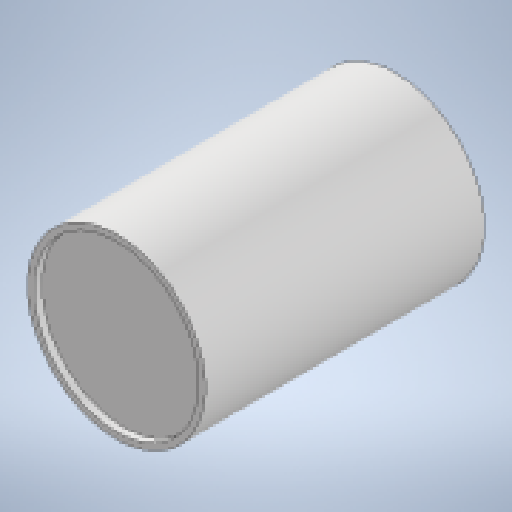
# Autodesk Inventor part: GrundkörperOben
Saved by Autodesk Inventor 2024 (Build 280153000, 153)
## iProperties
Created: 2024-02-13
Part Number: GrundkörperOben
Material: Generic
Document SubType Name: Modeling
Designer: Daniel Nussbaum
Density: 1 g/cm^3
Appearance: Default
Author: Daniel Nussbaum
Autodesk Inventor part; units mm, degrees
ref_plane "YZ Plane" through (0, 0, 0) normal (1, 0, 0) x (0, 1, 0)
ref_plane "XZ Plane" through (0, 0, 0) normal (0, 1, 0) x (-1, 0, 0)
ref_plane "XY Plane" through (0, 0, 0) normal (0, 0, 1) x (1, 0, 0)
sketch "Sketch1" plane through (0, 0, 0) normal (0, 1, 0) x (-1, 0, 0)
  line L0 (-67.5, -60) -> (-67.5, 0)
  line L1 (2.5, -60) -> (2.5, 0)
  line L2 (-67.5, 0) -> (2.5, 0)
  line L3 (-32.5, 0) -> (-32.5, 110)
  line L4 (2.5, -60) -> (-67.5, -60) projected
  line L5 (-67.5, 0) -> (-67.5, 110)
  line L6 (-65, 0) -> (-65, -30)
  line L7 (0, 0) -> (0, -30)
  line L8 (-65, 0) -> (-65, 110)
  line L9 (-65, 110) -> (-67.5, 110)
  line L10 (-65, 0) -> (-67.5, 0)
  line L11 (-65, 107) -> (-32.5, 107)
  line L12 (-32.5, 107) -> (-32.5, 102)
  line L13 (-32.5, 102) -> (-65, 102)
  line L14 (-65, 102) -> (-65, 107)
  dimension "d1" = 170
  dimension "d2" = 5
  dimension "d3" = 3
  constraints: 28 end point, 7 vertical, 3 parallel, 2 horizontal, 2 perpendicular, 2 point on line, 1 midpoint, 7 other
  measures "d1" distance from line of L3.end L4
  measures "d2" distance between parallel lines of L11 L13
  measures "d3" distance between parallel lines of L9 L11
revolve "Revolution1" add sketch "Sketch1" angle 360 about axis through (32.5, 0, 0) along (0, 0, 1) contours L5 L9 L8 L2 | L8 L11 L3 L13
sketch "Sketch2" plane through (0, 0, 0) normal (0, 1, 0) x (-1, 0, 0)
  line L0 (2.5, 0) -> (-67.5, 0) projected
  line L1 (2.5, 110) -> (-67.5, 110) projected
  line L2 (-32.5, 0) -> (-32.5, 5)
  circle A0 centre (-32.5, 5) radius 1.5
  point P0 (0, 0)
  dimension "d5" = 5
  dimension "d6" = 3
  constraints: 2 end point, 1 centre point, 1 coincident, 1 midpoint, 1 vertical
  measures "d5" distance of L2.start L2.end
  measures "d6" diameter of A0
extrude "Extrusion1" cut sketch "Sketch2" along normal through all both and the other way through all
sketch "Sketch3" plane through (0, 0, 0) normal (1, 0, 0) x (0, 1, 0)
  line L0 (35, 0) -> (-35, 0) projected
  line L1 (35, 110) -> (-35, 110) projected
  line L2 (0, 0) -> (0, 5)
  circle A0 centre (0, 5) radius 1.5
  point P0 (34.9678, 5)
  point P1 (-34.9678, 5)
  dimension "d9" = 5
  dimension "d10" = 3
  constraints: 2 end point, 1 centre point, 1 coincident, 1 vertical
  measures "d9" distance of L2.start L2.end
  measures "d10" diameter of A0
extrude "Extrusion2" cut sketch "Sketch3" along normal through all both and the other way through all
body "Solid1"
